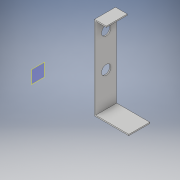
# Autodesk Inventor part: Fixação sem Tanque_2 - DIN
Saved by Autodesk Inventor 2019 (Build 230136000, 136)
## iProperties
Created: 2015-09-14
Part Number: Fixação sem Tanque_2 - DIN
Material: Genérico
Document SubType Name: Modeling
Designer: BAJA UEA
Density: 1 g/cm^3
Appearance: Padrão
Mass: 4352.78 g
Surface Area: 3520.72 cm^2
Volume: 4352.78 cm^3
Author: BAJA UEA
Autodesk Inventor part; units mm, degrees
ref_plane "YZ Plane" through (0, 0, 0) normal (1, 0, 0) x (0, 1, 0)
ref_plane "XZ Plane" through (0, 0, 0) normal (0, 1, 0) x (-1, 0, 0)
ref_plane "XY Plane" through (0, 0, 0) normal (0, 0, 1) x (1, 0, 0)
ref_plane "Plano de trabalho5" through (-1094.0332, 113.1084, -225.312) normal (0, 1, 0) x (1, 0, 0)
sketch "Esboço10" plane through (-1094.0332, 113.1084, -225.312) normal (0, 1, 0) x (1, 0, 0)
  line L0 (115.9279, 81.534) -> (115.9279, 81.534)
  circle A0 centre (115.9279, -5.1435) radius 8.001
  circle A1 centre (115.9279, 52.6415) radius 8.001
  line L1 (98.0571, -16.7405) -> (133.6171, -16.7405)
  line L2 (133.6171, 68.072) -> (133.6171, 42.672)
  line L3 (133.6171, -16.7405) -> (98.0571, -16.7405)
  line L4 (98.0571, -16.7405) -> (98.0571, 99.695)
  line L5 (133.6171, 99.695) -> (133.6171, -16.7405)
  line L6 (98.0571, 99.695) -> (98.0571, 110.395)
  line L7 (98.0571, 110.395) -> (133.6171, 110.395)
  line L8 (133.6171, 110.395) -> (133.6171, 99.695)
  line L9 (133.6171, 110.395) -> (98.0571, 110.395)
  line L10 (98.0571, 110.395) -> (98.0571, -16.7405)
  line L11 (98.0571, -16.7405) -> (133.6171, -16.7405)
  line L12 (133.6171, -16.7405) -> (133.6171, 110.395)
  point P0 (1094.0332, -225.312)
  dimension "d30" = 0
  dimension "d35" = 16.002
  dimension "d37" = 16.002
  dimension "d65" = 10.7
  constraints: 26 end point, 4 parallel, 3 horizontal, 2 centre point, 2 perpendicular
  measures "d30" distance of L0.start L0.end
  measures "d35" diameter of A0
  measures "d37" diameter of A1
  measures "d65" distance of L6.start L6.end
extrude "Extrusão9" add sketch "Esboço10" along normal blind 2
sketch "Esboço14" plane through (-960.416, 113.1084, -335.707) normal (0, 0, -1) x (-1, 0, 0)
  line L0 (0, 2) -> (35.56, 2)
  line L1 (35.56, 2) -> (35.56, -18.1014)
  line L2 (0, -5.2428) -> (35.56, -18.1014)
  line L3 (0, -5.2428) -> (0, 2)
  point P0 (-960.416, -113.1084)
  constraints: 8 end point, 1 horizontal, 1 perpendicular, 1 vertical
extrude "Extrusão12" add sketch "Esboço14" along normal blind 2
sketch "Esboço15" plane through (-960.416, 113.1084, -335.707) normal (0, 0, 1) x (1, 0, 0)
  line L0 (-35.56, -18.1014) -> (-35.56, 2) projected
  line L1 (0, 2) -> (0, -5.2428) projected
  line L2 (-35.56, -18.1014) -> (0, -5.2428)
  line L3 (0, -5.2428) -> (0, -18.1014)
  line L4 (0, -18.1014) -> (-35.56, -18.1014)
  point P0 (960.416, -113.1084)
  constraints: 6 end point, 1 collinear, 1 perpendicular
extrude "Extrusão13" add sketch "Esboço15" against normal blind 2.0066
sketch "Esboço16" plane through (-960.416, 113.1084, -335.707) normal (0, 0, 1) x (1, 0, 0)
  line L0 (-35.56, -18.1014) -> (-35.56, 2) projected
  line L1 (-35.56, -18.1014) -> (0, -18.1014)
  line L2 (0, -18.1014) -> (0, -56.2014)
  line L3 (0, -56.2014) -> (-35.56, -56.2014)
  line L4 (-35.56, -56.2014) -> (-35.56, -18.1014)
  point P0 (960.416, -113.1084)
  dimension "d70" = 38.1
  constraints: 8 end point, 2 parallel, 1 horizontal, 1 perpendicular
  measures "d70" distance of L1.end L2.end
extrude "Extrusão14" add sketch "Esboço16" against normal blind 2.0066
sketch "Esboço17" plane through (-995.976, 113.1084, -208.5715) normal (0, 0, 1) x (1, 0, 0)
  line L0 (35.56, 0) -> (35.56, 2) projected
  line L1 (0, 0) -> (0, 2) projected
  line L2 (35.56, 0) -> (0, 0)
  line L3 (0, 0) -> (0, 2)
  line L4 (0, 2) -> (35.56, 2)
  line L5 (35.56, 2) -> (35.56, 0)
  point P0 (995.976, -113.1084)
  constraints: 8 end point, 2 parallel, 1 horizontal, 1 perpendicular
extrude "Extrusão15" add sketch "Esboço17" along normal blind 12.7
sketch "Esboço18" plane through (-1094.0332, 113.1084, -225.312) normal (0, -1, 0) x (1, 0, 0)
  line L0 (98.0571, 29.4405) -> (133.6171, 29.4405) projected
  line L1 (133.6171, 29.4405) -> (133.6171, -110.395) projected
  line L2 (98.0571, 29.4405) -> (133.6171, 29.4405)
  line L3 (133.6171, 29.4405) -> (133.6171, 27.4339)
  line L4 (133.6171, 27.4339) -> (98.0571, 27.4339)
  line L5 (98.0571, 27.4339) -> (98.0571, 29.4405)
  point P0 (1094.0332, 225.312)
  dimension "d75" = 2.0066
  constraints: 8 end point, 2 parallel, 1 horizontal, 1 perpendicular, 1 point on line
  measures "d75" distance of L2.end L3.end
extrude "Extrusão16" add sketch "Esboço18" along normal blind 17.9832
body "Solid1"
